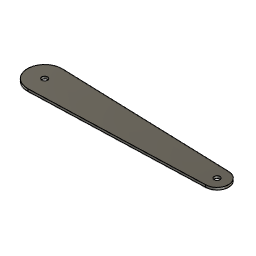
BRAZO v4 (Autodesk Fusion 360 design; units mm, degrees)
Autodesk Fusion 360 part; units mm, degrees
note: some values were not read from the file. Set by a fixed rule: which sketch regions a step uses.
sketch "Boceto1" plane through (0, 0, 0) normal (0, 0, 1) x (1, 0, 0)
  circle A0 centre (0, 0) radius 30
  circle A1 centre (300, 0) radius 20
  line L0 (-0.001, 30) -> (300.6656, 19.9889)
  line L1 (300, -20) -> (1.0011, -29.9833)
  circle A2 centre (300, 0) radius 5
  circle A3 centre (0, 0) radius 5
  line L2 (0, 0) -> (50, 0)
  line L3 (50, 0) -> (100, 0)
  line L4 (150, 0) -> (200, 0)
  line L5 (100, 0) -> (150, 0)
  line L6 (250, 0) -> (300, 0)
  line L7 (200, 0) -> (250, 0)
  line L8 (0, 0) -> (-15, 0)
  constraint coincident A0.centre A3.centre
  constraint coincident A0 L0.start
  constraint coincident A1 L0.end
  constraint tangent A1 L0
  constraint coincident A1 L1.start
  constraint coincident A0 L1.end
  constraint tangent A0 L1
  constraint concentric A1 A2
  constraint horizontal L2
  constraint parallel L2 L3
  constraint horizontal L5
  constraint parallel L4 L5
  constraint horizontal L7
  constraint parallel L6 L7
  constraint horizontal L8
extrude "Extruir2" add sketch "Boceto1" along normal blind 4 contours A0 L0 | A0 A1 L1 L2 L3 L4 L5 L6 L7 | A0 A1 L0 L2 L3 L4 L5 L6 L7 | A1 picked at (-1.5634, 21.558)
extrude "Extruir1" [suppressed]
